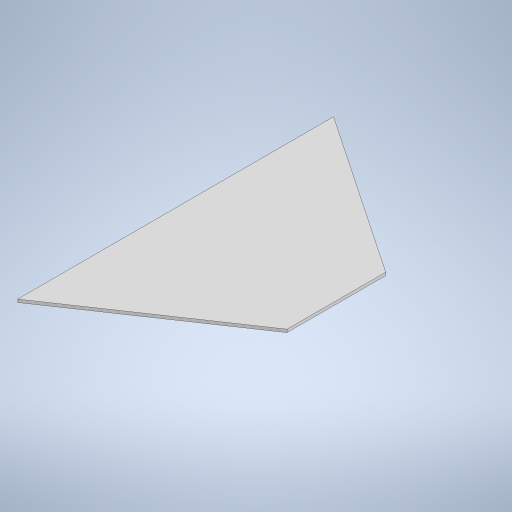
# Autodesk Inventor part: FLU-SidePlatesRS3
Saved by Autodesk Inventor 2024.3 (Build 283343000, 343)
## iProperties
Created: 2025-06-13
Part Number: FLU-SidePlatesRS3
Material: Generic
Document SubType Name: Modeling
Designer: ajclo
Density: 1 g/cm^3
Appearance: Default
Author: ajclo
Autodesk Inventor part; units mm, degrees
ref_plane "YZ Plane" through (0, 0, 0) normal (1, 0, 0) x (0, 1, 0)
ref_plane "XZ Plane" through (0, 0, 0) normal (0, 1, 0) x (-1, 0, 0)
ref_plane "XY Plane" through (0, 0, 0) normal (0, 0, 1) x (1, 0, 0)
sketch "Sketch1" plane through (0, 0, 0) normal (0, 1, 0) x (-1, 0, 0)
  line L0 (-81.4325, 160) -> (81.4325, 160)
  line L1 (81.4325, 160) -> (81.4325, -160)
  line L2 (81.4325, -160) -> (-81.4325, -160)
  line L3 (-81.4325, -160) -> (-81.4325, 160)
  line L4 (-81.4325, 160) -> (81.4325, -160) construction
  line L5 (81.4325, 160) -> (-81.4325, -160) construction
  line L6 (81.4325, 160) -> (-81.4325, 50)
  line L7 (81.4325, -160) -> (-81.4325, -50)
  point P0 (0, 0)
  dimension "d0" = 320
  dimension "d1" = 162.865
  dimension "d2" = 100
  dimension "d3" = 50
  constraints: 16 end point, 2 midpoint, 2 parallel, 2 point on line, 1 horizontal, 1 perpendicular
  measures "d0" distance of L0.end L1.end
  measures "d1" distance of L1.end L2.end
  measures "d2" distance of L6.end L7.end
  measures "d3" vertical distance of point (0, 0) L6.end
extrude "Extrusion1" add sketch "Sketch1" along normal blind 3 contours L1 L7 L3 L6
body "Solid1"
